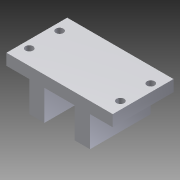
# Autodesk Inventor part: 8020_sliders
Saved by Autodesk Inventor 2011 (Build 150239000, 239)
## iProperties
Created: 2013-01-17
Part Number: 8020_sliders
Document SubType Name: Modeling
Designer: Christopher
Density: 1 g/cm^3
Author: Christopher
Autodesk Inventor part; units mm, degrees
ref_plane "YZ Plane" through (0, 0, 0) normal (1, 0, 0) x (0, 1, 0)
ref_plane "XZ Plane" through (0, 0, 0) normal (0, 1, 0) x (-1, 0, 0)
ref_plane "XY Plane" through (0, 0, 0) normal (0, 0, 1) x (1, 0, 0)
sketch "Sketch1" plane through (0, 0, 0) normal (0, 0, 1) x (1, 0, 0)
  line L0 (-50.7247, 3.2468) -> (38.1753, 3.2468)
  line L1 (38.1753, 3.2468) -> (38.1753, -6.2782)
  line L2 (-50.7247, -6.2782) -> (-50.7247, 3.2468)
  line L3 (38.1753, -6.2782) -> (19.1253, -6.2782)
  line L4 (-50.7247, -6.2782) -> (-31.6747, -6.2782)
  line L5 (-31.6747, -6.2782) -> (-31.6747, -31.6782)
  line L6 (19.1253, -6.2782) -> (19.1253, -31.6782)
  line L7 (19.1253, -31.6782) -> (6.4253, -31.6782)
  line L8 (-31.6747, -31.6782) -> (-18.9747, -31.6782)
  line L9 (-18.9747, -31.6782) -> (-18.9747, -6.2782)
  line L10 (-18.9747, -6.2782) -> (6.4253, -6.2782)
  line L11 (6.4253, -6.2782) -> (6.4253, -31.6782)
  point P0 (0, 0)
  dimension "d0" = 88.9
  dimension "d1" = 9.525
  dimension "d2" = 19.05
  dimension "d3" = 19.05
  dimension "d4" = 25.4
  dimension "d5" = 12.7
  dimension "d6" = 12.7
  constraints: 24 end point, 5 perpendicular, 4 parallel, 2 collinear, 1 horizontal
  measures "d0" distance of L0.start L0.end
  measures "d1" distance of L0.end L1.end
  measures "d2" distance of L1.end L3.end
  measures "d3" distance of L2.start L4.end
  measures "d4" distance of L4.end L5.end
  measures "d5" distance of L6.end L7.end
  measures "d6" distance of L5.end L8.end
extrude "Extrusion1" add sketch "Sketch1" against normal blind 50.8
sketch "Sketch2" plane through (-50.7247, 3.2468, 0) normal (0, 1, 0) x (1, 0, 0)
  line L0 (88.9, 50.8) -> (0, 50.8) projected
  line L1 (0, 0) -> (88.9, 0) projected
  line L2 (88.9, 0) -> (88.9, 50.8) projected
  line L3 (44.45, 0) -> (44.45, 50.8)
  point P0 (50.7247, 0)
  point P1 (82.55, 12.7)
  point P2 (82.55, 38.1)
  point P3 (6.35, 38.1)
  point P4 (6.35, 12.7)
  dimension "d9" = 44.45
  dimension "d10" = 38.1
  dimension "d11" = 38.1
  dimension "d12" = 38.1
  dimension "d13" = 38.1
  dimension "d14" = 25.4
  dimension "d15" = 25.4
  dimension "d16" = 12.7
  dimension "d17" = 12.7
  constraints: 2 end point, 2 midpoint, 1 perpendicular
  measures "d9" distance between parallel lines of L2 L3
  measures "d10" distance from line of L3 point (82.55, 12.7)
  measures "d11" distance from line of L3 point (82.55, 38.1)
  measures "d12" distance from line of point (6.35, 38.1) L3
  measures "d13" distance from line of L3 point (6.35, 12.7)
  measures "d14" distance of point (6.35, 38.1) point (6.35, 12.7)
  measures "d15" distance of point (82.55, 38.1) point (82.55, 12.7)
  measures "d16" distance from line of L1 point (82.55, 12.7)
  measures "d17" distance from line of L1 point (6.35, 12.7)
hole "Hole1" at (31.8253, 3.2468, -12.7) at (31.8253, 3.2468, -38.1) at (-44.3747, 3.2468, -38.1) at (-44.3747, 3.2468, -12.7) direction (0, -1, 0) diameter 6.35 depth 25.4 tip angle 118
body "Solid1"
